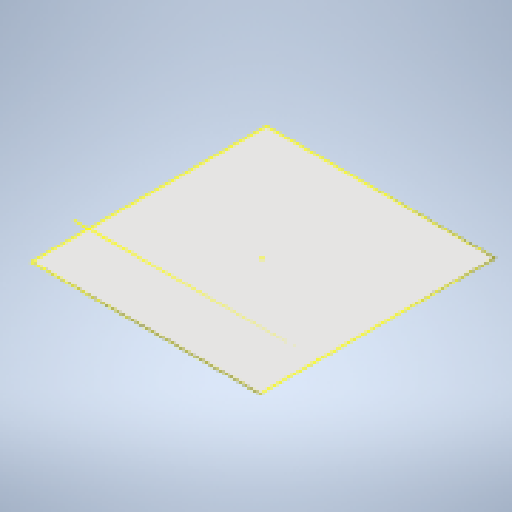
# Autodesk Inventor part: inclind sheet2
Saved by Autodesk Inventor 2025.2 (Build 292293000, 293)
## iProperties
Created: 2025-05-26
Part Number: inclind sheet2
Material: Generic
Document SubType Name: Sheet Metal
Designer: abdal
Density: 1 g/cm^3
Sheet Metal Rule: Default_mm
Appearance: Default
Author: abdal
Autodesk Inventor part; units mm, degrees
ref_plane "YZ Plane" through (0, 0, 0) normal (1, 0, 0) x (0, 1, 0)
ref_plane "XZ Plane" through (0, 0, 0) normal (0, 1, 0) x (-1, 0, 0)
ref_plane "XY Plane" through (0, 0, 0) normal (0, 0, 1) x (1, 0, 0)
sketch "Sketch1" plane through (0, 0, 0) normal (0, 1, 0) x (-1, 0, 0)
  line L0 (510, 515) -> (-510, 515)
  line L1 (-510, 515) -> (-510, -515)
  line L2 (-510, -515) -> (510, -515)
  line L3 (510, -515) -> (510, 515)
  line L4 (510, 515) -> (-510, -515) construction
  line L5 (-510, 515) -> (510, -515) construction
  point P0 (0, 0)
  dimension "d0" = 1020
  dimension "d1" = 1030
  measures "d0" distance of L1.end L2.end
  measures "d1" distance of L0.end L1.end
extrude "Plate1" add sketch "Sketch1" along normal blind 2
sketch "Sketch2" plane through (0, 0, 0) normal (0, -1, 0) x (1, 0, 0)
  line L0 (-492.0259, 515) -> (-492.0259, -515) projected
  line L1 (510, 515) -> (510, -515) projected
  line L2 (-510, 515) -> (510, 515) projected
  line L3 (-510, -515) -> (-510, 515) projected
  line L4 (510, -515) -> (-510, -515) projected
  point P0 (0, 0)
extrude "Extrusion1" cut sketch "Sketch2" against normal through all contours L0 L4 L3 L2
sketch "Sketch3" plane through (0, 2, 0) normal (0, 1, 0) x (1, 0, 0)
  line L0 (509.927, -255.216) -> (502.87, -255.6841) projected
  line L1 (-555.9699, -264.6411) -> (509.927, -255.216) projected
  line L2 (-492.0259, 515) -> (-492.0259, -515) projected
  line L3 (510, -515) -> (-492.0259, -515) projected
  line L4 (510, 515) -> (510, -515) projected
  line L5 (-492.0259, 515) -> (510, 515) projected
  line L6 (509.927, -255.216) -> (510, -255.216)
  point P0 (0, 0)
  point P1 (-492.0259, -264.0757)
  constraints: 2 end point, 1 perpendicular, 1 point on line
extrude "Extrusion2" cut sketch "Sketch3" against normal through all contours L1 L6 L4 L3 L2
sketch "Sketch4" plane through (0, 2, 0) normal (0, 1, 0) x (1, 0, 0)
  line L0 (-492.0259, -264.0757) -> (-492.0259, 515) projected
  line L1 (-492.0259, -264.0757) -> (-572.0259, -264.0757)
  line L2 (-572.0259, -264.0757) -> (-572.0259, 515)
  line L3 (-572.0259, 515) -> (-492.0259, 515)
  line L4 (-492.0259, 515) -> (-492.0259, -264.0757)
  point P0 (0, 0)
  point P1 (-532.0259, 515)
  point P2 (-492.0259, 515)
  dimension "d7" = 80
  dimension "d8" = 740.457
  constraints: 8 end point, 2 parallel, 1 horizontal, 1 midpoint, 1 perpendicular
  measures "d7" distance of L2.end L3.end
  measures "d8" distance of point (0, 0) point (-532.026, 515)
extrude "Extrusion3" add sketch "Sketch4" against normal blind 2
equation "\"d2\" = Thickness"
equation "\"BendRadius\" = Thickness"
equation "\"BendReliefWidth\" = Thickness"
equation "\"BendReliefDepth\" = 0.5 * Thickness"
equation "\"CornerReliefSize\" = 4 * Thickness"
equation "\"MinimumRemnant\" = 2 * Thickness"
equation "\"TransitionRadius\" = BendRadius"
equation "\"JacobiRadiusSize\" = BendRadius"
equation "\"GapSize\" = Thickness"
equation "\"Thickness\" = 2"
body "Solid1"
